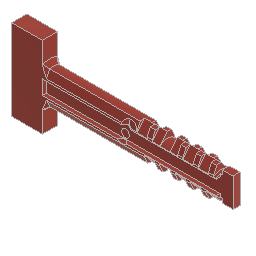
protec (Autodesk Fusion 360 design; units mm, degrees)
Autodesk Fusion 360 part; units mm, degrees
note: some values were not read from the file. Chosen so that the rebuilt part matches the saved one: which face or edge a step refers to; where a step starts; which pieces of a blend or face edit are solid. Set by a fixed rule: which sketch regions a step uses.
sketch "base/0 cut" plane through (0, 0, 0) normal (1, 0, 0) x (0, 1, 0)
  line L0 (0, 0) -> (3.3, 0) construction
  line L1 (3.3, 0) -> (3.3, 3.3) construction
  line L2 (3.3, 3.3) -> (4, 3.3) construction
  line L3 (4, 3.3) -> (4, 4.7)
  line L4 (4, 4.7) -> (4.775, 4.7)
  line L5 (4.775, 4.7) -> (4.775, 5.1226)
  line L6 (4.775, 5.1226) -> (4.1363, 6.4923)
  line L7 (4.775, 5.1226) -> (1.825, 5.1226) construction
  line L8 (3.3, 3.3) -> (2.6, 3.3) construction
  line L9 (2.6, 3.3) -> (2.6, 4.7)
  line L10 (2.6, 4.7) -> (1.825, 4.7)
  line L11 (1.825, 4.7) -> (1.825, 5.1226)
  line L12 (1.825, 5.1226) -> (2.4637, 6.4923)
  line L13 (1.825, 5.1226) -> (4.775, 5.1226) construction
  arc A0 (4.1363, 6.4923) -> (2.4637, 6.4923) centre (3.3, 3.3) ccw
  line L14 (2.6, 3.3) -> (2.6, 1.9)
  line L15 (2.6, 1.9) -> (1.825, 1.9)
  line L16 (1.825, 1.9) -> (1.825, 1.4774)
  line L17 (1.825, 1.4774) -> (2.4637, 0.1077)
  line L18 (1.825, 1.4774) -> (4.775, 1.4774) construction
  line L19 (4, 3.3) -> (4, 1.9)
  line L20 (4, 1.9) -> (4.775, 1.9)
  line L21 (4.775, 1.9) -> (4.775, 1.4774)
  line L22 (4.775, 1.4774) -> (4.1363, 0.1077)
  line L23 (4.775, 1.4774) -> (1.825, 1.4774) construction
  arc A1 (2.4637, 0.1077) -> (4.1363, 0.1077) centre (3.3, 3.3) ccw
  circle A2 centre (3.3, 3.3) radius 3.7125
  dimension "d27" = 3.3
  dimension "d28" = 3.3
  dimension "d29" = 0.7
  dimension "d30" = 1.4
  dimension "d31" = 0.775
  dimension "d32" = 0.4226
  dimension "d33" = 65
  dimension "d34" = 1.5113
  dimension "d35" = 0.7
  dimension "d36" = 1.4
  dimension "d37" = 0.775
  dimension "d38" = 0.4226
  dimension "d39" = 65
  dimension "d40" = 1.5113
  dimension "d41" = 1.4
  dimension "d42" = 0.775
  dimension "d43" = 0.4226
  dimension "d44" = 1.5113
  dimension "d45" = 65
  dimension "d46" = 1.4
  dimension "d47" = 0.775
  dimension "d48" = 0.4226
  dimension "d49" = 65
  dimension "d50" = 1.5113
  dimension "d51" = 7.425
  constraint coincident L0.start origin
  constraint horizontal L0
  constraint perpendicular L0 L1
  constraint perpendicular L1 L2
  constraint perpendicular L2 L3
  constraint perpendicular L3 L4
  constraint perpendicular L4 L5
  constraint horizontal L7
  constraint perpendicular L1 L8
  constraint perpendicular L8 L9
  constraint perpendicular L9 L10
  constraint perpendicular L10 L11
  constraint horizontal L13
  constraint coincident L1.end L2.start
  constraint perpendicular L8 L14
  constraint perpendicular L14 L15
  constraint perpendicular L15 L16
  constraint horizontal L18
  constraint perpendicular L2 L19
  constraint perpendicular L19 L20
  constraint perpendicular L20 L21
  constraint horizontal L23
  constraint concentric A1 A2
  measures "d27" distance of L0.start L0.end
  measures "d28" distance of L0.end L1.end
  measures "d29" distance of L1.end L2.end
  measures "d30" distance of L2.end L3.end
  measures "d31" distance of L3.end L4.end
  measures "d32" distance of L4.end L5.end
  measures "d33" angle of L6 L7
  measures "d34" distance of L5.end L6.end
  measures "d35" distance of L1.end L8.end
  measures "d36" distance of L8.end L9.end
  measures "d37" distance of L9.end L10.end
  measures "d38" distance of L10.end L7.end
  measures "d39" angle of L12 L13
  measures "d40" distance of L7.end L12.end
  measures "d41" distance of L8.end L14.end
  measures "d42" distance of L14.end L15.end
  measures "d43" distance of L15.end L16.end
  measures "d44" distance of L16.end L17.end
  measures "d45" angle of L17 L18
  measures "d46" distance of L2.end L19.end
  measures "d47" distance of L19.end L20.end
  measures "d48" distance of L20.end L18.end
  measures "d49" angle of L22 L23
  measures "d50" distance of L18.end L22.end
  measures "d51" diameter of A2
extrude "Extrude1" add sketch "base/0 cut" against normal blind 42.57 contours L3 L4 L5 L6 L9 L10 L11 L12 A0 L14 L15 L16 L17 L19 L20 L21 L22 A1 makes body 1
sketch "dss holes" plane through (0, 2.6, 0) normal (0, -1, 0) x (1, 0, 0)
  line L0 (0, 1.9) -> (0, 4.7)
  line L1 (0, 4.7) -> (-42.57, 4.7)
  line L2 (-42.57, 4.7) -> (-42.57, 1.9)
  line L3 (-42.57, 1.9) -> (0, 1.9)
  line L4 (0, 3.3) -> (-19.57, 3.3) construction
  line L5 (-19.57, 3.3) -> (-16.57, 3.3) construction
  line L6 (-19.57, 3.3) -> (-19.57, 4.9) construction
  line L7 (-19.57, 3.3) -> (-19.57, 1.7) construction
  line L8 (-16.57, 3.3) -> (-16.57, 4.9) construction
  line L9 (-16.57, 3.3) -> (-16.57, 1.7) construction
  circle A0 centre (-19.57, 4.9) radius 0.9
  circle A1 centre (-19.57, 1.7) radius 0.9
  circle A2 centre (-16.57, 4.9) radius 0.9
  circle A3 centre (-16.57, 1.7) radius 0.9
  line L10 (-19.57, 3.3) -> (-21.07, 3.3) construction
  line L11 (-21.07, 3.3) -> (-21.07, 2.5) construction
  line L12 (-21.07, 3.3) -> (-21.07, 4.1) construction
  dimension "d54" = 19.57
  dimension "d55" = 3
  dimension "d56" = 1.6
  dimension "d57" = 1.6
  dimension "d58" = 1.6
  dimension "d59" = 1.6
  dimension "d60" = 1.8
  dimension "d61" = 1.8
  dimension "d62" = 1.8
  dimension "d63" = 1.8
  dimension "d64" = 1.5
  dimension "d65" = 0.8
  dimension "d66" = 0.8
  constraint midpoint L0 L4.start
  constraint perpendicular L0 L4
  constraint parallel L4 L5
  constraint perpendicular L5 L6
  constraint perpendicular L4 L7
  constraint perpendicular L4 L8
  constraint perpendicular L4 L9
  constraint coincident L6.end A0.centre
  constraint coincident L7.end A1.centre
  constraint coincident L8.end A2.centre
  constraint coincident L9.end A3.centre
  constraint perpendicular L7 L10
  constraint perpendicular L10 L11
  constraint perpendicular L10 L12
  measures "d54" distance of L4.start L4.end
  measures "d55" distance of L4.end L5.end
  measures "d56" distance of L4.end L6.end
  measures "d57" distance of L4.end L7.end
  measures "d58" distance of L5.end L8.end
  measures "d59" distance of L5.end L9.end
  measures "d60" diameter of A0
  measures "d61" diameter of A1
  measures "d62" diameter of A2
  measures "d63" diameter of A3
  measures "d64" distance of L4.end L10.end
  measures "d65" distance of L10.end L11.end
  measures "d66" distance of L10.end L12.end
extrude "Extrude18" cut sketch "dss holes" along normal blind 0.9 draft 35 from surface at -0.125 contours L1 A0 | L1 A0 bodies 1
extrude "Extrude19" cut sketch "dss holes" against normal blind 0.9 draft 35 from surface at -1.275 contours L3 A1 | L3 A1 bodies 1
sketch "dc holes" plane through (0, 0, 0) normal (1, 0, 0) x (0, 1, 0)
  line L0 (0, 0) -> (3.3, 0) construction
  line L1 (3.3, 0) -> (3.3, 3.3) construction
  line L2 (3.3, 3.3) -> (-1.6893, 2.056) construction
  line L3 (3.3, 3.3) -> (-1.7, 3.3) construction
  line L4 (3.3, 3.3) -> (-1.7, 3.3) construction
  line L5 (3.3, 3.3) -> (1.4542, 2.8398) construction
  circle A0 centre (1.4542, 2.8398) radius 1.375
  line L6 (3.3, 3.3) -> (8.3, 3.3) construction
  line L7 (3.3, 3.3) -> (8.2893, 4.544) construction
  line L8 (3.3, 3.3) -> (8.3, 3.3) construction
  line L9 (3.3, 3.3) -> (5.1458, 3.7602) construction
  circle A1 centre (5.1458, 3.7602) radius 1.375
  dimension "d223" = 3.3
  dimension "d224" = 3.3
  dimension "d225" = 14
  dimension "d226" = 5.1421
  dimension "d227" = 5
  dimension "d228" = 1.9023
  dimension "d229" = 2.75
  dimension "d230" = 5
  dimension "d231" = 5.1421
  dimension "d232" = 14
  dimension "d233" = 1.9023
  dimension "d234" = 2.75
  constraint coincident L0.start origin
  constraint horizontal L0
  constraint perpendicular L0 L1
  constraint horizontal L3
  constraint perpendicular L1 L4
  constraint parallel L2 L5
  constraint coincident L5.end A0.centre
  constraint perpendicular L1 L6
  constraint horizontal L8
  constraint parallel L7 L9
  constraint coincident L9.end A1.centre
  measures "d223" distance of L0.start L0.end
  measures "d224" distance of L0.end L1.end
  measures "d225" angle of L2 L3
  measures "d226" distance of L1.end L2.end
  measures "d227" distance of L1.end L3.end
  measures "d228" distance of L1.end L5.end
  measures "d229" diameter of A0
  measures "d230" distance of L1.end L6.end
  measures "d231" distance of L1.end L7.end
  measures "d232" angle of L7 L8
  measures "d233" distance of L1.end L9.end
  measures "d234" diameter of A1
extrude "Extrude17" add sketch "dc holes" along normal mid plane 2.75 separate body makes body 2 at (0.9167, 6.5191, 3.6917) makes body 3 at (0.9167, 2.8275, 2.7712)
fillet "Fillet1" radius 1.375 4 edges at (-1.375, 3.8639, 4.2574) (1.375, 3.8639, 3.263) (1.375, 0.1722, 2.3426) (-1.375, 0.1722, 3.337) on bodies 2 3
move_body "MoveFace1" bodies 2 3 to x (1, 0, 0) y (0, 1, 0) z (0, 0, 1) at (-21.07, 0, 0) on bodies 2 3
combine "Combine1" operation cut target body 1 tool bodies 2 3
sketch "bow" plane through (-42.57, 0, 0) normal (-1, 0, 0) x (0, -1, 0)
  line L0 (-2.6, 1.9) -> (-2.6, 4.7)
  line L1 (-2.6, 4.7) -> (-1.825, 4.7)
  line L2 (-1.825, 4.7) -> (-1.825, 5.1226)
  line L3 (-1.825, 5.1226) -> (-2.4637, 6.4923)
  arc A0 (-2.4637, 6.4923) -> (-4.1363, 6.4923) centre (-3.3, 3.3) ccw
  line L4 (-4.1363, 6.4923) -> (-4.775, 5.1226)
  line L5 (-4.775, 5.1226) -> (-4.775, 4.7)
  line L6 (-4.775, 4.7) -> (-4, 4.7)
  line L7 (-4, 4.7) -> (-4, 1.9)
  line L8 (-4, 1.9) -> (-4.775, 1.9)
  line L9 (-4.775, 1.9) -> (-4.775, 1.4774)
  line L10 (-4.775, 1.4774) -> (-4.1363, 0.1077)
  arc A1 (-4.1363, 0.1077) -> (-2.4637, 0.1077) centre (-3.3, 3.3) ccw
  line L11 (-2.4637, 0.1077) -> (-1.825, 1.4774)
  line L12 (-1.825, 1.4774) -> (-1.825, 1.9)
  line L13 (-1.825, 1.9) -> (-2.6, 1.9)
  line L14 (-4.775, 1.9) -> (-4.775, 4.7)
  circle A2 centre (-3.3, 3.3) radius 3.3 construction
  line L15 (-1.825, 1.9) -> (-1.825, 4.7)
  line L16 (-1.825, 4.7) -> (-1.825, 6.252)
  line L17 (-1.825, 1.9) -> (-1.825, 0.348)
  line L18 (-4.775, 1.9) -> (-4.775, 0.348)
  line L19 (-4.775, 4.7) -> (-4.775, 6.252)
  line L20 (-1.825, 6.252) -> (-1.825, 11.252)
  line L21 (-4.775, 6.252) -> (-4.775, 11.252)
  line L22 (-4.775, 11.252) -> (-1.825, 11.252)
  line L23 (-4.775, 0.348) -> (-4.775, -4.652)
  line L24 (-1.825, 0.348) -> (-1.825, -4.652)
  line L25 (-4.775, -4.652) -> (-1.825, -4.652)
  dimension "d67" = 6.6
  dimension "d68" = 5
  dimension "d69" = 5
  dimension "d70" = 5
  dimension "d71" = 5
  constraint coincident L8.end L9.start
  constraint coincident L5.end L6.start
  constraint concentric A0 A2
  constraint coincident L12.end L13.start
  constraint coincident L1.end L2.start
  constraint coincident A2 L16.end
  constraint parallel L2 L16
  constraint coincident A2 L17.end
  constraint perpendicular L13 L17
  constraint coincident A2 L18.end
  constraint parallel L9 L18
  constraint coincident A2 L19.end
  constraint parallel L5 L19
  constraint parallel L16 L20
  constraint parallel L19 L21
  constraint parallel L18 L23
  constraint parallel L17 L24
  measures "d67" diameter of A2
  measures "d68" distance of L16.end L20.end
  measures "d69" distance of L19.end L21.end
  measures "d70" distance of L18.end L23.end
  measures "d71" distance of L17.end L24.end
extrude "Extrude2" add sketch "bow" against normal blind 6 bodies 1
chamfer "Chamfer1" distance 0.8 angle 45 6 edges at (-36.57, 3.3, 6.6) (-36.57, 2.1443, 5.8074) (-36.57, 4.4557, 5.8074) (-36.57, 4.4557, 0.7926) (-36.57, 3.3, 0) (-36.57, 2.1443, 0.7926) on bodies 1
sketch "tip cut" plane through (0, 0, 0) normal (1, 0, 0) x (0, 1, 0)
  line L0 (0, 0) -> (3.3, 0) construction
  line L1 (3.3, 0) -> (3.3, 3.3) construction
  line L2 (3.3, 3.3) -> (4, 3.3) construction
  line L3 (3.3, 3.3) -> (2.6, 3.3) construction
  circle A0 centre (3.3, 3.3) radius 2.9 construction
  line L4 (4, 3.3) -> (4, 6.1142)
  line L5 (4, 3.3) -> (4, 0.4858)
  line L6 (2.6, 3.3) -> (2.6, 0.4858)
  line L7 (2.6, 3.3) -> (2.6, 6.1142)
  arc A1 (4, 6.1142) -> (2.6, 6.1142) centre (3.3, 3.3) ccw
  arc A2 (2.6, 0.4858) -> (4, 0.4858) centre (3.3, 3.3) ccw
  circle A3 centre (3.3, 3.3) radius 3.3
  dimension "d75" = 3.3
  dimension "d76" = 3.3
  dimension "d77" = 0.7
  dimension "d78" = 0.7
  dimension "d79" = 5.8
  dimension "d80" = 6.6
  constraint coincident L0.start origin
  constraint horizontal L0
  constraint perpendicular L0 L1
  constraint perpendicular L1 L2
  constraint perpendicular L1 L3
  constraint coincident L1.end L2.start
  constraint coincident A0 L4.end
  constraint perpendicular L2 L4
  constraint coincident A0 L5.end
  constraint perpendicular L2 L5
  constraint coincident A0 L6.end
  constraint perpendicular L3 L6
  constraint coincident A0 L7.end
  constraint perpendicular L3 L7
  constraint concentric A0 A3
  measures "d75" distance of L0.start L0.end
  measures "d76" distance of L0.end L1.end
  measures "d77" distance of L1.end L2.end
  measures "d78" distance of L1.end L3.end
  measures "d79" diameter of A0
  measures "d80" diameter of A3
sketch "1 cut" plane through (0, 0, 0) normal (1, 0, 0) x (0, 1, 0)
  line L0 (0, 0) -> (3.3, 0) construction
  line L1 (3.3, 0) -> (3.3, 3.3) construction
  line L2 (3.3, 3.3) -> (4, 3.3) construction
  line L3 (3.3, 3.3) -> (2.6, 3.3) construction
  line L4 (4, 3.3) -> (4, 4.7)
  line L5 (2.6, 3.3) -> (2.6, 4.7)
  line L6 (4, 4.7) -> (4.775, 4.7)
  line L7 (2.6, 4.7) -> (1.825, 4.7)
  line L8 (4.775, 4.7) -> (4.775, 4.8422)
  line L9 (1.825, 4.7) -> (1.825, 5.1226)
  line L10 (4.775, 4.8422) -> (3.3, 6.6)
  line L11 (4.775, 4.8422) -> (1.825, 4.8422) construction
  line L12 (1.825, 5.1226) -> (2.4637, 6.4923)
  line L13 (1.825, 5.1226) -> (4.5397, 5.1226) construction
  arc A0 (3.3, 6.6) -> (2.4637, 6.4923) centre (3.3, 3.3) ccw
  line L14 (4, 3.3) -> (4, 1.9)
  line L15 (2.6, 3.3) -> (2.6, 1.9)
  line L16 (4, 1.9) -> (4.775, 1.9)
  line L17 (2.6, 1.9) -> (1.825, 1.9)
  line L18 (1.825, 1.9) -> (1.825, 1.7578)
  line L19 (4.775, 1.9) -> (4.775, 1.4774)
  line L20 (1.825, 1.7578) -> (3.3, 0)
  line L21 (1.825, 1.7578) -> (4.775, 1.7578) construction
  line L22 (4.775, 1.4774) -> (4.1363, 0.1077)
  line L23 (4.775, 1.4774) -> (2.0603, 1.4774) construction
  arc A1 (3.3, 0) -> (4.1363, 0.1077) centre (3.3, 3.3) ccw
  circle A2 centre (3.3, 3.3) radius 3.7125
  dimension "d81" = 3.3
  dimension "d82" = 3.3
  dimension "d83" = 0.7
  dimension "d84" = 0.7
  dimension "d85" = 1.4
  dimension "d86" = 1.4
  dimension "d87" = 0.775
  dimension "d88" = 0.775
  dimension "d89" = 0.1422
  dimension "d90" = 0.4226
  dimension "d91" = 50
  dimension "d92" = 2.2947
  dimension "d93" = 65
  dimension "d94" = 1.5113
  dimension "d95" = 3.3
  dimension "d96" = 1.4
  dimension "d97" = 1.4
  dimension "d98" = 0.775
  dimension "d99" = 0.775
  dimension "d100" = 0.1422
  dimension "d101" = 0.4226
  dimension "d102" = 2.2947
  dimension "d103" = 50
  dimension "d104" = 65
  dimension "d105" = 1.5113
  dimension "d106" = 3.3
  dimension "d107" = 7.425
  constraint coincident L0.start origin
  constraint horizontal L0
  constraint perpendicular L0 L1
  constraint perpendicular L1 L2
  constraint perpendicular L1 L3
  constraint perpendicular L2 L4
  constraint perpendicular L3 L5
  constraint perpendicular L4 L6
  constraint perpendicular L5 L7
  constraint perpendicular L6 L8
  constraint perpendicular L7 L9
  constraint horizontal L11
  constraint coincident L9 L11.end
  constraint horizontal L13
  constraint coincident L10 L13.end
  constraint perpendicular L2 L14
  constraint perpendicular L3 L15
  constraint perpendicular L14 L16
  constraint perpendicular L15 L17
  constraint perpendicular L17 L18
  constraint perpendicular L16 L19
  constraint horizontal L21
  constraint coincident L19 L21.end
  constraint horizontal L23
  constraint coincident L20 L23.end
  constraint concentric A0 A2
  measures "d81" distance of L0.start L0.end
  measures "d82" distance of L0.end L1.end
  measures "d83" distance of L1.end L2.end
  measures "d84" distance of L1.end L3.end
  measures "d85" distance of L2.end L4.end
  measures "d86" distance of L3.end L5.end
  measures "d87" distance of L4.end L6.end
  measures "d88" distance of L5.end L7.end
  measures "d89" distance of L6.end L8.end
  measures "d90" distance of L7.end L9.end
  measures "d91" angle of L10 L11
  measures "d92" distance of L8.end L10.end
  measures "d93" angle of L12 L13
  measures "d94" distance of L9.end L12.end
  measures "d95" radius of A0
  measures "d96" distance of L2.end L14.end
  measures "d97" distance of L3.end L15.end
  measures "d98" distance of L14.end L16.end
  measures "d99" distance of L15.end L17.end
  measures "d100" distance of L17.end L18.end
  measures "d101" distance of L16.end L19.end
  measures "d102" distance of L18.end L0.end
  measures "d103" angle of L20 L21
  measures "d104" angle of L22 L23
  measures "d105" distance of L19.end L22.end
  measures "d106" radius of A1
  measures "d107" diameter of A2
sketch "2 cut" plane through (0, 0, 0) normal (1, 0, 0) x (0, 1, 0)
  line L0 (0, 0) -> (3.3, 0) construction
  line L1 (3.3, 0) -> (3.3, 3.3) construction
  line L2 (3.3, 3.3) -> (4, 3.3) construction
  line L3 (3.3, 3.3) -> (2.6, 3.3) construction
  line L4 (4, 3.3) -> (4, 4.7)
  line L5 (2.6, 3.3) -> (2.6, 4.7)
  line L6 (2.6, 3.3) -> (2.6, 1.9)
  line L7 (4, 3.3) -> (4, 1.9)
  line L8 (4, 4.7) -> (4.775, 4.7)
  line L9 (2.6, 4.7) -> (1.825, 4.7)
  line L10 (4, 1.9) -> (4.775, 1.9)
  line L11 (2.6, 1.9) -> (1.825, 1.9)
  line L12 (1.825, 4.7) -> (1.825, 4.8422)
  line L13 (4.775, 1.9) -> (4.775, 1.7578)
  line L14 (1.825, 1.9) -> (1.825, 1.4774)
  line L15 (4.775, 4.7) -> (4.775, 5.1226)
  line L16 (1.825, 4.8422) -> (3.3, 6.6)
  line L17 (1.825, 4.8422) -> (4.775, 4.8422) construction
  line L18 (4.775, 5.1226) -> (4.1363, 6.4923)
  line L19 (4.775, 5.1226) -> (2.0603, 5.1226) construction
  arc A0 (4.1363, 6.4923) -> (3.3, 6.6) centre (3.3, 3.3) ccw
  line L20 (4.775, 1.7578) -> (3.3, 0)
  line L21 (4.775, 1.7578) -> (1.825, 1.7578) construction
  line L22 (1.825, 1.4774) -> (2.4637, 0.1077)
  line L23 (1.825, 1.4774) -> (4.5397, 1.4774) construction
  arc A1 (2.4637, 0.1077) -> (3.3, 0) centre (3.3, 3.3) ccw
  circle A2 centre (3.3, 3.3) radius 3.7125
  dimension "d108" = 3.3
  dimension "d109" = 3.3
  dimension "d110" = 0.7
  dimension "d111" = 0.7
  dimension "d112" = 1.4
  dimension "d113" = 1.4
  dimension "d114" = 1.4
  dimension "d115" = 1.4
  dimension "d116" = 0.775
  dimension "d117" = 0.775
  dimension "d118" = 0.775
  dimension "d119" = 0.775
  dimension "d120" = 0.1422
  dimension "d121" = 0.1422
  dimension "d122" = 0.4226
  dimension "d123" = 0.4226
  dimension "d124" = 2.2947
  dimension "d125" = 50
  dimension "d126" = 65
  dimension "d127" = 1.5113
  dimension "d128" = 3.3
  dimension "d129" = 50
  dimension "d130" = 2.2947
  dimension "d131" = 65
  dimension "d132" = 1.5113
  dimension "d133" = 3.3
  dimension "d134" = 7.425
  constraint coincident L0.start origin
  constraint horizontal L0
  constraint perpendicular L0 L1
  constraint perpendicular L1 L2
  constraint perpendicular L1 L3
  constraint perpendicular L2 L4
  constraint perpendicular L3 L5
  constraint perpendicular L3 L6
  constraint perpendicular L2 L7
  constraint perpendicular L4 L8
  constraint perpendicular L5 L9
  constraint perpendicular L7 L10
  constraint perpendicular L6 L11
  constraint perpendicular L9 L12
  constraint perpendicular L10 L13
  constraint perpendicular L11 L14
  constraint perpendicular L8 L15
  constraint horizontal L17
  constraint coincident L15 L17.end
  constraint horizontal L19
  constraint coincident L16 L19.end
  constraint horizontal L21
  constraint coincident L14 L21.end
  constraint horizontal L23
  constraint coincident L20 L23.end
  constraint concentric A1 A2
  measures "d108" distance of L0.start L0.end
  measures "d109" distance of L0.end L1.end
  measures "d110" distance of L1.end L2.end
  measures "d111" distance of L1.end L3.end
  measures "d112" distance of L2.end L4.end
  measures "d113" distance of L3.end L5.end
  measures "d114" distance of L3.end L6.end
  measures "d115" distance of L2.end L7.end
  measures "d116" distance of L4.end L8.end
  measures "d117" distance of L5.end L9.end
  measures "d118" distance of L7.end L10.end
  measures "d119" distance of L6.end L11.end
  measures "d120" distance of L9.end L12.end
  measures "d121" distance of L10.end L13.end
  measures "d122" distance of L11.end L14.end
  measures "d123" distance of L8.end L15.end
  measures "d124" distance of L12.end L16.end
  measures "d125" angle of L16 L17
  measures "d126" angle of L18 L19
  measures "d127" distance of L15.end L18.end
  measures "d128" radius of A0
  measures "d129" angle of L20 L21
  measures "d130" distance of L13.end L0.end
  measures "d131" angle of L22 L23
  measures "d132" distance of L14.end L22.end
  measures "d133" radius of A1
  measures "d134" diameter of A2
sketch "3 cut" plane through (0, 0, 0) normal (1, 0, 0) x (0, 1, 0)
  line L0 (0, 0) -> (3.3, 0) construction
  line L1 (3.3, 0) -> (3.3, 3.3) construction
  line L2 (3.3, 3.3) -> (4, 3.3) construction
  line L3 (3.3, 3.3) -> (2.6, 3.3) construction
  line L4 (4, 3.3) -> (4, 4.7)
  line L5 (4, 3.3) -> (4, 1.9)
  line L6 (2.6, 3.3) -> (2.6, 1.9)
  line L7 (2.6, 3.3) -> (2.6, 4.7)
  line L8 (4, 4.7) -> (4.775, 4.7)
  line L9 (2.6, 4.7) -> (1.825, 4.7)
  line L10 (4, 1.9) -> (4.775, 1.9)
  line L11 (2.6, 1.9) -> (1.825, 1.9)
  line L12 (4.775, 4.7) -> (4.775, 4.8422)
  line L13 (1.825, 4.7) -> (1.825, 5.1226)
  line L14 (4.775, 1.9) -> (4.775, 1.4774)
  line L15 (1.825, 1.9) -> (1.825, 1.7578)
  line L16 (4.775, 4.8422) -> (3.1292, 5.9946)
  line L17 (4.775, 4.8422) -> (1.825, 4.8422) construction
  line L18 (1.825, 5.1226) -> (2.1038, 5.7206)
  line L19 (1.825, 5.1226) -> (4.3745, 5.1226) construction
  arc A0 (3.1292, 5.9946) -> (2.1038, 5.7206) centre (3.3, 3.3) ccw
  line L20 (1.825, 1.7578) -> (3.4708, 0.6054)
  line L21 (1.825, 1.7578) -> (4.775, 1.7578) construction
  line L22 (4.775, 1.4774) -> (4.4962, 0.8794)
  line L23 (4.775, 1.4774) -> (2.2255, 1.4774) construction
  arc A1 (3.4708, 0.6054) -> (4.4962, 0.8794) centre (3.3, 3.3) ccw
  circle A2 centre (3.3, 3.3) radius 3.7125
  dimension "d135" = 3.3
  dimension "d136" = 3.3
  dimension "d137" = 0.7
  dimension "d138" = 0.7
  dimension "d139" = 1.4
  dimension "d140" = 1.4
  dimension "d141" = 1.4
  dimension "d142" = 1.4
  dimension "d143" = 0.775
  dimension "d144" = 0.775
  dimension "d145" = 0.775
  dimension "d146" = 0.775
  dimension "d147" = 0.1422
  dimension "d148" = 0.4226
  dimension "d149" = 0.4226
  dimension "d150" = 0.1422
  dimension "d151" = 35
  dimension "d152" = 2.0092
  dimension "d153" = 0.6598
  dimension "d154" = 65
  dimension "d155" = 2.7
  dimension "d156" = 2.0092
  dimension "d157" = 35
  dimension "d158" = 65
  dimension "d159" = 0.6598
  dimension "d160" = 2.7
  dimension "d161" = 7.425
  constraint coincident L0.start origin
  constraint horizontal L0
  constraint perpendicular L0 L1
  constraint perpendicular L1 L2
  constraint perpendicular L1 L3
  constraint perpendicular L2 L4
  constraint perpendicular L2 L5
  constraint perpendicular L3 L6
  constraint perpendicular L3 L7
  constraint perpendicular L4 L8
  constraint perpendicular L7 L9
  constraint perpendicular L5 L10
  constraint perpendicular L6 L11
  constraint perpendicular L8 L12
  constraint perpendicular L9 L13
  constraint perpendicular L10 L14
  constraint perpendicular L11 L15
  constraint horizontal L17
  constraint coincident L13 L17.end
  constraint horizontal L19
  constraint coincident L16 L19.end
  constraint horizontal L21
  constraint coincident L14 L21.end
  constraint horizontal L23
  constraint coincident L20 L23.end
  constraint concentric A0 A2
  measures "d135" distance of L0.start L0.end
  measures "d136" distance of L0.end L1.end
  measures "d137" distance of L1.end L2.end
  measures "d138" distance of L1.end L3.end
  measures "d139" distance of L2.end L4.end
  measures "d140" distance of L2.end L5.end
  measures "d141" distance of L3.end L6.end
  measures "d142" distance of L3.end L7.end
  measures "d143" distance of L4.end L8.end
  measures "d144" distance of L7.end L9.end
  measures "d145" distance of L5.end L10.end
  measures "d146" distance of L6.end L11.end
  measures "d147" distance of L8.end L12.end
  measures "d148" distance of L9.end L13.end
  measures "d149" distance of L10.end L14.end
  measures "d150" distance of L11.end L15.end
  measures "d151" angle of L16 L17
  measures "d152" distance of L12.end L16.end
  measures "d153" distance of L13.end L18.end
  measures "d154" angle of L18 L19
  measures "d155" radius of A0
  measures "d156" distance of L15.end L20.end
  measures "d157" angle of L20 L21
  measures "d158" angle of L22 L23
  measures "d159" distance of L14.end L22.end
  measures "d160" radius of A1
  measures "d161" diameter of A2
sketch "4 cut" plane through (0, 0, 0) normal (1, 0, 0) x (0, 1, 0)
  line L0 (0, 0) -> (3.3, 0) construction
  line L1 (3.3, 0) -> (3.3, 3.3) construction
  line L2 (3.3, 3.3) -> (4, 3.3) construction
  line L3 (3.3, 3.3) -> (2.6, 3.3) construction
  line L4 (4, 3.3) -> (4, 4.7)
  line L5 (4, 3.3) -> (4, 1.9)
  line L6 (2.6, 3.3) -> (2.6, 4.7)
  line L7 (2.6, 3.3) -> (2.6, 1.9)
  line L8 (4, 4.7) -> (4.775, 4.7)
  line L9 (2.6, 4.7) -> (1.825, 4.7)
  line L10 (4, 1.9) -> (4.775, 1.9)
  line L11 (2.6, 1.9) -> (1.825, 1.9)
  line L12 (4.775, 4.7) -> (4.775, 4.8422)
  line L13 (1.825, 4.7) -> (1.825, 4.8422)
  line L14 (1.825, 1.9) -> (1.825, 1.7578)
  line L15 (4.775, 1.9) -> (4.775, 1.7578)
  line L16 (4.775, 4.8422) -> (3.8512, 5.9431)
  line L17 (4.775, 4.8422) -> (1.825, 4.8422) construction
  line L18 (1.825, 4.8422) -> (2.7488, 5.9431)
  line L19 (1.825, 4.8422) -> (4.775, 4.8422) construction
  arc A0 (3.8512, 5.9431) -> (2.7488, 5.9431) centre (3.3, 3.3) ccw
  line L20 (4.775, 1.7578) -> (3.8512, 0.6569)
  line L21 (4.775, 1.7578) -> (1.825, 1.7578) construction
  line L22 (1.825, 1.7578) -> (2.7488, 0.6569)
  line L23 (1.825, 1.7578) -> (4.775, 1.7578) construction
  arc A1 (2.7488, 0.6569) -> (3.8512, 0.6569) centre (3.3, 3.3) ccw
  circle A2 centre (3.3, 3.3) radius 3.7125
  dimension "d162" = 3.3
  dimension "d163" = 3.3
  dimension "d164" = 0.7
  dimension "d165" = 0.7
  dimension "d166" = 1.4
  dimension "d167" = 1.4
  dimension "d168" = 1.4
  dimension "d169" = 1.4
  dimension "d170" = 0.775
  dimension "d171" = 0.775
  dimension "d172" = 0.775
  dimension "d173" = 0.775
  dimension "d174" = 0.1422
  dimension "d175" = 0.1422
  dimension "d176" = 0.1422
  dimension "d177" = 0.1422
  dimension "d178" = 50
  dimension "d179" = 1.4372
  dimension "d180" = 50
  dimension "d181" = 1.4372
  dimension "d182" = 50
  dimension "d183" = 1.4372
  dimension "d184" = 50
  dimension "d185" = 1.4372
  dimension "d186" = 7.425
  constraint coincident L0.start origin
  constraint horizontal L0
  constraint perpendicular L0 L1
  constraint perpendicular L1 L2
  constraint perpendicular L1 L3
  constraint perpendicular L2 L4
  constraint perpendicular L2 L5
  constraint perpendicular L3 L6
  constraint perpendicular L3 L7
  constraint perpendicular L4 L8
  constraint perpendicular L6 L9
  constraint perpendicular L5 L10
  constraint perpendicular L7 L11
  constraint perpendicular L8 L12
  constraint perpendicular L9 L13
  constraint perpendicular L11 L14
  constraint perpendicular L10 L15
  constraint horizontal L17
  constraint horizontal L19
  constraint coincident L1.end L2.start
  constraint horizontal L21
  constraint horizontal L23
  constraint concentric A1 A2
  measures "d162" distance of L0.start L0.end
  measures "d163" distance of L0.end L1.end
  measures "d164" distance of L1.end L2.end
  measures "d165" distance of L1.end L3.end
  measures "d166" distance of L2.end L4.end
  measures "d167" distance of L2.end L5.end
  measures "d168" distance of L3.end L6.end
  measures "d169" distance of L3.end L7.end
  measures "d170" distance of L4.end L8.end
  measures "d171" distance of L6.end L9.end
  measures "d172" distance of L5.end L10.end
  measures "d173" distance of L7.end L11.end
  measures "d174" distance of L8.end L12.end
  measures "d175" distance of L9.end L13.end
  measures "d176" distance of L11.end L14.end
  measures "d177" distance of L10.end L15.end
  measures "d178" angle of L16 L17
  measures "d179" distance of L12.end L16.end
  measures "d180" angle of L18 L19
  measures "d181" distance of L13.end L18.end
  measures "d182" angle of L20 L21
  measures "d183" distance of L15.end L20.end
  measures "d184" angle of L22 L23
  measures "d185" distance of L14.end L22.end
  measures "d186" diameter of A2
sketch "5 cut" plane through (0, 0, 0) normal (1, 0, 0) x (0, 1, 0)
  line L0 (0, 0) -> (3.3, 0) construction
  line L1 (3.3, 0) -> (3.3, 3.3) construction
  line L2 (3.3, 3.3) -> (4, 3.3) construction
  line L3 (3.3, 3.3) -> (2.6, 3.3) construction
  line L4 (4, 3.3) -> (4, 4.7)
  line L5 (4, 3.3) -> (4, 1.9)
  line L6 (2.6, 3.3) -> (2.6, 4.7)
  line L7 (2.6, 3.3) -> (2.6, 1.9)
  line L8 (4, 4.7) -> (4.775, 4.7)
  line L9 (2.6, 4.7) -> (1.825, 4.7)
  line L10 (4, 1.9) -> (4.775, 1.9)
  line L11 (2.6, 1.9) -> (1.825, 1.9)
  line L12 (1.825, 4.7) -> (1.825, 4.8422)
  line L13 (4.775, 4.7) -> (4.775, 5.1226)
  line L14 (1.825, 1.9) -> (1.825, 1.4774)
  line L15 (4.775, 1.9) -> (4.775, 1.7578)
  line L16 (1.825, 4.8422) -> (3.4708, 5.9946)
  line L17 (1.825, 4.8422) -> (4.775, 4.8422) construction
  line L18 (4.775, 5.1226) -> (4.4962, 5.7206)
  line L19 (4.775, 5.1226) -> (2.2255, 5.1226) construction
  arc A0 (4.4962, 5.7206) -> (3.4708, 5.9946) centre (3.3, 3.3) ccw
  line L20 (4.775, 1.7578) -> (3.1292, 0.6054)
  line L21 (4.775, 1.7578) -> (1.825, 1.7578) construction
  line L22 (1.825, 1.4774) -> (2.1038, 0.8794)
  line L23 (1.825, 1.4774) -> (4.3745, 1.4774) construction
  arc A1 (2.1038, 0.8794) -> (3.1292, 0.6054) centre (3.3, 3.3) ccw
  circle A2 centre (3.3, 3.3) radius 3.7125
  dimension "d187" = 3.3
  dimension "d188" = 3.3
  dimension "d189" = 0.7
  dimension "d190" = 0.7
  dimension "d191" = 1.4
  dimension "d192" = 1.4
  dimension "d193" = 1.4
  dimension "d194" = 1.4
  dimension "d195" = 0.775
  dimension "d196" = 0.775
  dimension "d197" = 0.775
  dimension "d198" = 0.775
  dimension "d199" = 0.1422
  dimension "d200" = 0.4226
  dimension "d201" = 0.4226
  dimension "d202" = 0.1422
  dimension "d203" = 35
  dimension "d204" = 2.0092
  dimension "d205" = 65
  dimension "d206" = 0.6598
  dimension "d207" = 2.7
  dimension "d208" = 35
  dimension "d209" = 2.0092
  dimension "d210" = 0.6598
  dimension "d211" = 65
  dimension "d212" = 2.7
  dimension "d213" = 7.425
  constraint coincident L0.start origin
  constraint horizontal L0
  constraint perpendicular L0 L1
  constraint perpendicular L1 L2
  constraint perpendicular L1 L3
  constraint perpendicular L2 L4
  constraint perpendicular L2 L5
  constraint perpendicular L3 L6
  constraint perpendicular L3 L7
  constraint perpendicular L4 L8
  constraint perpendicular L6 L9
  constraint perpendicular L5 L10
  constraint perpendicular L7 L11
  constraint perpendicular L9 L12
  constraint perpendicular L8 L13
  constraint perpendicular L11 L14
  constraint perpendicular L10 L15
  constraint horizontal L17
  constraint coincident L13 L17.end
  constraint horizontal L19
  constraint coincident L16 L19.end
  constraint horizontal L21
  constraint coincident L14 L21.end
  constraint horizontal L23
  constraint coincident L20 L23.end
  constraint concentric A0 A2
  measures "d187" distance of L0.start L0.end
  measures "d188" distance of L0.end L1.end
  measures "d189" distance of L1.end L2.end
  measures "d190" distance of L1.end L3.end
  measures "d191" distance of L2.end L4.end
  measures "d192" distance of L2.end L5.end
  measures "d193" distance of L3.end L6.end
  measures "d194" distance of L3.end L7.end
  measures "d195" distance of L4.end L8.end
  measures "d196" distance of L6.end L9.end
  measures "d197" distance of L5.end L10.end
  measures "d198" distance of L7.end L11.end
  measures "d199" distance of L9.end L12.end
  measures "d200" distance of L8.end L13.end
  measures "d201" distance of L11.end L14.end
  measures "d202" distance of L10.end L15.end
  measures "d203" angle of L16 L17
  measures "d204" distance of L12.end L16.end
  measures "d205" angle of L18 L19
  measures "d206" distance of L13.end L18.end
  measures "d207" radius of A0
  measures "d208" angle of L20 L21
  measures "d209" distance of L15.end L20.end
  measures "d210" distance of L14.end L22.end
  measures "d211" angle of L22 L23
  measures "d212" radius of A1
  measures "d213" diameter of A2
sketch "6 cut" plane through (0, 0, 0) normal (1, 0, 0) x (0, 1, 0)
  line L0 (0, 0) -> (3.3, 0) construction
  line L1 (3.3, 0) -> (3.3, 3.3) construction
  line L2 (3.3, 3.3) -> (4, 3.3) construction
  line L3 (4, 3.3) -> (4, 4.7) construction
  line L4 (4, 4.7) -> (4.775, 4.7) construction
  line L5 (4.775, 4.7) -> (4.775, 4.8422) construction
  line L6 (4.775, 4.8422) -> (3.1292, 5.9946) construction
  line L7 (4.775, 4.8422) -> (1.861, 4.8422) construction
  circle A0 centre (3.3, 3.3) radius 2.1093
  circle A1 centre (3.3, 3.3) radius 3.7125
  dimension "d214" = 3.3
  dimension "d215" = 3.3
  dimension "d216" = 0.7
  dimension "d217" = 1.4
  dimension "d218" = 0.775
  dimension "d219" = 0.1422
  dimension "d220" = 35
  dimension "d221" = 2.0092
  dimension "d222" = 7.425
  constraint coincident L0.start origin
  constraint horizontal L0
  constraint perpendicular L0 L1
  constraint perpendicular L1 L2
  constraint perpendicular L2 L3
  constraint perpendicular L3 L4
  constraint perpendicular L4 L5
  constraint horizontal L7
  constraint coincident L1.end L2.start
  constraint tangent L6 A0
  constraint coincident L7.end A0
  constraint concentric A0 A1
  measures "d214" distance of L0.start L0.end
  measures "d215" distance of L0.end L1.end
  measures "d216" distance of L1.end L2.end
  measures "d217" distance of L2.end L3.end
  measures "d218" distance of L3.end L4.end
  measures "d219" distance of L4.end L5.end
  measures "d220" angle of L6 L7
  measures "d221" distance of L5.end L6.end
  measures "d222" diameter of A1
extrude "Extrude3" cut sketch "tip cut" against normal blind 2.57 bodies 1
extrude "Extrude4" cut sketch "6 cut" along normal mid plane 1 from surface at -2.57 bodies 1
extrude "1" cut sketch "1 cut" along normal mid plane 2 from surface at -3.57 bodies 1
extrude "2" cut sketch "2 cut" along normal mid plane 2 from surface at -5.07 bodies 1
extrude "3" cut sketch "1 cut" along normal mid plane 2 from surface at -6.57 bodies 1
extrude "4" cut sketch "2 cut" along normal mid plane 2 from surface at -8.07 bodies 1
extrude "5" cut sketch "1 cut" along normal mid plane 2 from surface at -9.57 bodies 1
extrude "6" cut sketch "2 cut" along normal mid plane 2 from surface at -11.07 bodies 1
extrude "7" cut sketch "6 cut" along normal mid plane 2 from surface at -12.57 bodies 1
extrude "8" cut sketch "2 cut" along normal mid plane 2 from surface at -14.07 bodies 1
extrude "9" cut sketch "1 cut" along normal mid plane 2 from surface at -15.57 bodies 1
extrude "10" cut sketch "2 cut" along normal mid plane 2 from surface at -17.07 bodies 1
equation "key_width = 2.95 mm"
equation "half_key_width = 0.5 * key_width"
equation "radius_one = 3.3 mm"
equation "radius_two = 2.7 mm"
equation "zero_disk_angle = 65 deg"
equation "one_two_disk_angle = zero_disk_angle - 15 deg"
equation "three_five_disk_angle = one_two_disk_angle - 15 deg"
equation "uncut_diagonal_width = 4.25 mm"
equation "half_key_side_height = ( 0.5 * 2.8 ) * 1 mm"
equation "zero_disk_height_full = 0.5 * ( ( ( ( uncut_diagonal_width / cos(90 deg - zero_disk_angle) ) ^ 2 ) - ( key_width ^ 2 ) ) ^ 0.5 )"
equation "zero_disk_height_partial = zero_disk_height_full - half_key_side_height"
equation "cut_height_full = ( radius_one ) - ( half_key_width / tan(40 deg) )"
equation "cut_height_partial = cut_height_full - half_key_side_height"
equation "a = -half_key_width"
equation "b1 = zero_disk_height_full"
equation "b2 = cut_height_full"
equation "x1 = ( -2 * tan(zero_disk_angle) * ( b1 - a * tan(zero_disk_angle) ) + sqrt(( 2 * tan(zero_disk_angle) * ( b1 - a * tan(zero_disk_angle) ) ) ^ 2 - 4 * ( 1 + ( tan(zero_disk_angle) ) ^ 2 ) * ( ( b1 - a * tan(zero_disk_angle) ) ^ 2 - radius_one ^ 2 )) ) / ( 2 * ( 1 + ( tan(zero_disk_angle) ) ^ 2 ) )"
equation "zero_cut_side_height = sqrt(( x1 - a ) ^ 2 + ( x1 * tan(zero_disk_angle) + b1 - a * tan(zero_disk_angle) - b1 ) ^ 2)"
equation "x2 = ( -2 * tan(three_five_disk_angle) * ( b2 - a * tan(three_five_disk_angle) ) + sqrt(( 2 * tan(three_five_disk_angle) * ( b2 - a * tan(three_five_disk_angle) ) ) ^ 2 - 4 * ( 1 + ( tan(three_five_disk_angle) ) ^ 2 ) * ( ( b2 - a * tan(three_five_disk_angle) ) ^ 2 - radius_two ^ 2 )) ) / ( 2 * ( 1 + ( tan(three_five_disk_angle) ) ^ 2 ) )"
equation "three_five_cut_side_height = sqrt(( x2 - a ) ^ 2 + ( x2 * tan(three_five_disk_angle) + b2 - a * tan(three_five_disk_angle) - b2 ) ^ 2)"
equation "x3 = ( -2 * tan(one_two_disk_angle) * ( b2 - a * tan(one_two_disk_angle) ) + sqrt(( 2 * tan(one_two_disk_angle) * ( b2 - a * tan(one_two_disk_angle) ) ) ^ 2 - 4 * ( 1 + ( tan(one_two_disk_angle) ) ^ 2 ) * ( ( b2 - a * tan(one_two_disk_angle) ) ^ 2 - radius_two ^ 2 )) ) / ( 2 * ( 1 + ( tan(one_two_disk_angle) ) ^ 2 ) )"
equation "four_cut_side_heigth = sqrt(( x3 - a ) ^ 2 + ( x3 * tan(one_two_disk_angle) + b2 - a * tan(one_two_disk_angle) - b2 ) ^ 2)"
equation "x4 = ( -2 * tan(one_two_disk_angle) * ( b2 - a * tan(one_two_disk_angle) ) + sqrt(( 2 * tan(one_two_disk_angle) * ( b2 - a * tan(one_two_disk_angle) ) ) ^ 2 - 4 * ( 1 + ( tan(one_two_disk_angle) ) ^ 2 ) * ( ( b2 - a * tan(one_two_disk_angle) ) ^ 2 - radius_one ^ 2 )) ) / ( 2 * ( 1 + ( tan(one_two_disk_angle) ) ^ 2 ) )"
equation "one_two_cut_side_heigth = sqrt(( x4 - a ) ^ 2 + ( x4 * tan(one_two_disk_angle) + b2 - a * tan(one_two_disk_angle) - b2 ) ^ 2)"
equation "x5 = ( -2 * tan(zero_disk_angle) * ( b1 - a * tan(zero_disk_angle) ) + sqrt(( 2 * tan(zero_disk_angle) * ( b1 - a * tan(zero_disk_angle) ) ) ^ 2 - 4 * ( 1 + ( tan(zero_disk_angle) ) ^ 2 ) * ( ( b1 - a * tan(zero_disk_angle) ) ^ 2 - radius_two ^ 2 )) ) / ( 2 * ( 1 + ( tan(zero_disk_angle) ) ^ 2 ) )"
equation "zero_cut_three_five_side_height = sqrt(( x5 - a ) ^ 2 + ( x5 * tan(zero_disk_angle) + b1 - a * tan(zero_disk_angle) - b1 ) ^ 2)"
equation "d27 = radius_one"
equation "d28 = radius_one"
equation "d29 = half_key_width - 0.775 mm"
equation "d30 = half_key_side_height"
equation "d31 = half_key_width - d29"
equation "d32 = zero_disk_height_partial"
equation "d33 = zero_disk_angle"
equation "d34 = zero_cut_side_height"
equation "d35 = d29"
equation "d36 = d30"
equation "d37 = d31"
equation "d38 = d32"
equation "d39 = d33"
equation "d40 = d34"
equation "d41 = d30"
equation "d42 = d31"
equation "d43 = d32"
equation "d44 = d34"
equation "d45 = d33"
equation "d46 = d30"
equation "d47 = d31"
equation "d48 = d32"
equation "d49 = d33"
equation "d50 = d34"
equation "d51 = 2.25 * radius_one"
equation "d52 = -( 2.57 mm + 35 mm + 2 mm + 3 mm )"
equation "d54 = 19.17 mm + 0.4 mm"
equation "d57 = d56"
equation "d58 = d56"
equation "d59 = d56"
equation "d61 = d60"
equation "d62 = d60"
equation "d63 = d60"
equation "d66 = d65"
equation "d69 = d68"
equation "d70 = d68"
equation "d71 = d68"
equation "d75 = radius_one"
equation "d76 = radius_one"
equation "d77 = d29"
equation "d78 = d29"
equation "d80 = 2 * radius_one"
equation "d81 = radius_one"
equation "d82 = radius_one"
equation "d83 = d29"
equation "d84 = d29"
equation "d85 = d30"
equation "d86 = d30"
equation "d87 = d31"
equation "d88 = d31"
equation "d89 = cut_height_partial"
equation "d90 = zero_disk_height_partial"
equation "d91 = one_two_disk_angle"
equation "d92 = one_two_cut_side_heigth"
equation "d93 = zero_disk_angle"
equation "d94 = zero_cut_side_height"
equation "d96 = d30"
equation "d97 = d30"
equation "d98 = d31"
equation "d99 = d31"
equation "d100 = d89"
equation "d101 = d90"
equation "d102 = d92"
equation "d103 = d91"
equation "d104 = d93"
equation "d105 = d94"
equation "d107 = d51"
equation "d108 = radius_one"
equation "d109 = radius_one"
equation "d110 = d29"
equation "d111 = d29"
equation "d112 = d30"
equation "d113 = d30"
equation "d114 = d30"
equation "d115 = d30"
equation "d116 = d31"
equation "d117 = d31"
equation "d118 = d31"
equation "d119 = d31"
equation "d120 = d89"
equation "d121 = d89"
equation "d122 = d90"
equation "d123 = d90"
equation "d124 = d92"
equation "d125 = d91"
equation "d126 = d93"
equation "d127 = d94"
equation "d129 = d91"
equation "d130 = d92"
equation "d131 = d93"
equation "d132 = d94"
equation "d134 = d51"
equation "d135 = radius_one"
equation "d136 = radius_one"
equation "d137 = d29"
equation "d138 = d29"
equation "d139 = d30"
equation "d140 = d30"
equation "d141 = d30"
equation "d142 = d30"
equation "d143 = d31"
equation "d144 = d31"
equation "d145 = d31"
equation "d146 = d31"
equation "d147 = d89"
equation "d148 = d90"
equation "d149 = d90"
equation "d150 = d89"
equation "d151 = three_five_disk_angle"
equation "d152 = three_five_cut_side_height"
equation "d153 = zero_cut_three_five_side_height"
equation "d154 = zero_disk_angle"
equation "d156 = d152"
equation "d157 = d151"
equation "d158 = zero_disk_angle"
equation "d159 = zero_cut_three_five_side_height"
equation "d161 = d51"
equation "d162 = radius_one"
equation "d163 = radius_one"
equation "d164 = d29"
equation "d165 = d29"
equation "d166 = d30"
equation "d167 = d30"
equation "d168 = d30"
equation "d169 = d30"
equation "d170 = d31"
equation "d171 = d31"
equation "d172 = d31"
equation "d173 = d31"
equation "d174 = d89"
equation "d175 = d89"
equation "d176 = d89"
equation "d177 = d89"
equation "d178 = one_two_disk_angle"
equation "d179 = four_cut_side_heigth"
equation "d180 = one_two_disk_angle"
equation "d181 = four_cut_side_heigth"
equation "d182 = one_two_disk_angle"
equation "d183 = four_cut_side_heigth"
equation "d184 = one_two_disk_angle"
equation "d185 = four_cut_side_heigth"
equation "d186 = d51"
equation "d187 = radius_one"
equation "d188 = radius_one"
equation "d189 = d29"
equation "d190 = d29"
equation "d191 = d30"
equation "d192 = d30"
equation "d193 = d30"
equation "d194 = d30"
equation "d195 = d31"
equation "d196 = d31"
equation "d197 = d31"
equation "d198 = d31"
equation "d199 = d89"
equation "d200 = d90"
equation "d201 = d90"
equation "d202 = d89"
equation "d203 = three_five_disk_angle"
equation "d204 = three_five_cut_side_height"
equation "d205 = zero_disk_angle"
equation "d206 = zero_cut_three_five_side_height"
equation "d208 = d203"
equation "d209 = d204"
equation "d210 = d206"
equation "d211 = d205"
equation "d213 = d51"
equation "d214 = radius_one"
equation "d215 = radius_one"
equation "d216 = d29"
equation "d217 = d30"
equation "d218 = d31"
equation "d219 = d89"
equation "d220 = three_five_disk_angle"
equation "d221 = three_five_cut_side_height"
equation "d222 = d51"
equation "d223 = radius_one"
equation "d224 = radius_one"
equation "d226 = ( 5 / cos(13.5 deg) ) * 1 mm"
equation "d230 = d227"
equation "d231 = d226"
equation "d232 = d225"
equation "d233 = d228"
equation "d234 = d229"
equation "d240 = -2.07 mm - ( 1.5 * 1 mm )"
equation "d243 = -2.07 mm - ( 1.5 * 2 mm )"
equation "d246 = -2.07 mm - ( 1.5 * 3 mm )"
equation "d249 = -2.07 mm - ( 1.5 * 4 mm )"
equation "d252 = -2.07 mm - ( 1.5 * 5 mm )"
equation "d255 = -2.07 mm - ( 1.5 * 6 mm )"
equation "d258 = -2.07 mm - ( 1.5 * 7 mm )"
equation "d261 = -2.07 mm - ( 1.5 * 8 mm )"
equation "d264 = -2.07 mm - ( 1.5 * 9 mm )"
equation "d267 = -2.07 mm - ( 1.5 * 10 mm )"
equation "d276 = ( 0.5 * 2.75 ) * 1 mm"
equation "d279 = ( 0.5 * 2.75 ) * 1 mm"
named bodies: "blade", "dc dimple 1", "dc dimple 2"
